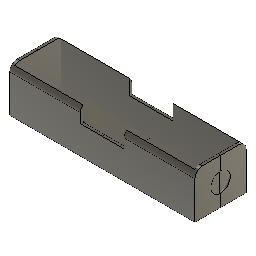
18620_holder v3 (Autodesk Fusion 360 design; units mm, degrees)
Autodesk Fusion 360 part; units mm, degrees
note: some values were not read from the file. Set by a fixed rule: which sketch regions a step uses.
sketch "Skizze1" plane through (0, 0, 0) normal (0, 0, 1) x (1, 0, 0)
  line L0 (0, 0) -> (38, 0)
  line L1 (38, 0) -> (38, 10.5)
  line L2 (38, 10.5) -> (0, 10.5)
  line L3 (0, 10.5) -> (0, 0)
  dimension "d1" = 38
  dimension "d2" = 10.5
  constraint horizontal L0
  constraint vertical L1
  constraint horizontal L2
  constraint vertical L3
  constraint coincident L0.start L3.end
  measures "d1" distance of L0.start L0.end
  measures "d2" distance of L0.end L1.end
extrude "Extrusion1" add sketch "Skizze1" along normal blind 18.5 makes body 1
shell "Schale1" thickness 1 removed faces 3 at (12.6667, 0, 6.1667) at (0, 3.5, 12.3333) at (25.3333, 3.5, 18.5) on bodies 1
fillet "Abrundung1" radius 3 1 edges at (19, 10.5, 18.5) on bodies 1
sketch "Skizze2" plane through (38, 0, 0) normal (1, 0, 0) x (0, 1, 0)
  arc A0 (10.5, 15.5) -> (7.5, 18.5) centre (7.5, 15.5) ccw
  line L0 (7.5, 18.5) -> (0, 18.5)
  line L1 (0, 18.5) -> (0, 0)
  line L2 (0, 0) -> (10.5, 0)
  line L3 (10.5, 0) -> (10.5, 15.5)
  circle A1 centre (0, 9) radius 4
  dimension "d8" = 9
  dimension "d9" = 8
  constraint coincident L1 A1.centre
  measures "d8" distance of L2 A1.centre
  measures "d9" diameter of A1
extrude "Extrusion2" cut sketch "Skizze2" against normal blind 0.5 contours L1 A1 picked at (1.594, 7.7807) bodies 1
sketch "Skizze3" plane through (0, 0, 18.5) normal (0, 0, 1) x (-1, 0, 0)
  line L0 (-38, -7.5) -> (-37, -7.5)
  line L1 (-37, -7.5) -> (-37, 0)
  line L2 (-37, 0) -> (-38, 0)
  line L3 (-38, 0) -> (-38, -7.5)
  line L4 (0, -9.5) -> (-9, -9.5)
  line L5 (-9, -9.5) -> (-9, -11.5)
  line L6 (-9, -11.5) -> (0, -11.5)
  line L7 (0, -11.5) -> (0, -9.5)
  line L8 (-37, 0) -> (0, 0)
  line L9 (0, 0) -> (0, -9.5)
  dimension "d12" = 9
  dimension "d13" = 2
  dimension "d14" = 9.5
  dimension "d16" = 29
  constraint horizontal L4
  constraint vertical L5
  constraint horizontal L6
  constraint vertical L7
  measures "d12" distance of L4.start L4.end
  measures "d13" distance of L4.end L5.end
  measures "d14" distance of L4 L8
  measures "d16" distance of L3 L5
extrude "Extrusion3" cut sketch "Skizze3" against normal blind 7 contours L4 L5 L6 L7 bodies 1
sketch "Skizze4" plane through (0, 0, 1) normal (0, 0, 1) x (-1, 0, 0)
  line L0 (0, -9.5) -> (0, 0)
  line L1 (0, 0) -> (-37, 0)
  line L2 (-37, 0) -> (-37, -9.5)
  line L3 (-37, -9.5) -> (0, -9.5)
  point P0 (-20, 0)
  dimension "d26" = 20
  constraint coincident L0.end L1.start
  constraint coincident L1 P0
  measures "d26" distance of L0.end P0
hole "Bohrung1" at (0, 0, 1) at (20, 0, 1) direction (0, 0, -1) diameter 3.2 depth 10 tip angle 118 bodies 1
mirror "Spiegeln1" about plane through (0, 0, 0) normal (0, 1, 0) of "Extrusion1", "Schale1", "Abrundung1", "Extrusion2", "Extrusion3", "Bohrung1" makes body 2
mirror "Spiegeln2" about plane through (0, 0, 0) normal (1, 0, 0) of "Extrusion1", "Schale1", "Abrundung1", "Extrusion2", "Extrusion3", "Bohrung1", "Spiegeln1" makes body 3 at (-27.6667, 9.5, 10.0787) makes body 4 at (-27.6667, -9.5, 10.0787)
equation "d1 = ( 76 / 2 ) * 1 mm"
equation "d2 = ( 21 / 2 ) * 1 mm"
equation "d16 = ( 76 / 2 ) * 1 mm - 9 mm"
